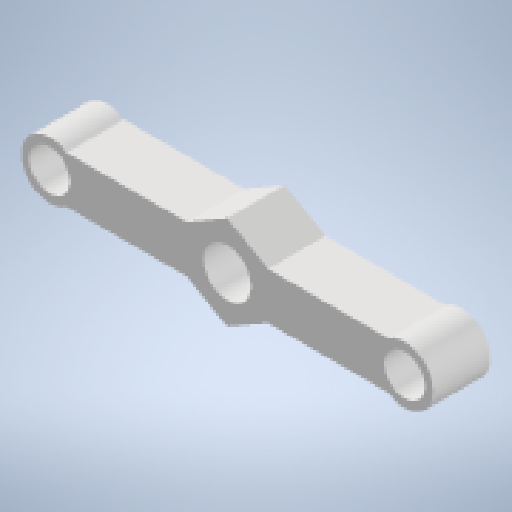
# Autodesk Inventor part: chep_za_os
Saved by Autodesk Inventor 2023 (Build 270158000, 158)
## iProperties
Created: 2022-09-29
Part Number: chep_za_os
Material: Generic
Document SubType Name: Modeling
Designer: simon
Density: 1 g/cm^3
Appearance: Default
Author: simon
Autodesk Inventor part; units mm, degrees
ref_plane "YZ Plane" through (0, 0, 0) normal (1, 0, 0) x (0, 1, 0)
ref_plane "XZ Plane" through (0, 0, 0) normal (0, 1, 0) x (-1, 0, 0)
ref_plane "XY Plane" through (0, 0, 0) normal (0, 0, 1) x (1, 0, 0)
sketch "Sketch1" plane through (0, 0, 0) normal (0, 0, 1) x (1, 0, 0)
  line L0 (0, -7.5) -> (-6.4952, -3.75) projected
  line L1 (-6.4952, -3.75) -> (-6.4952, 3.75) projected
  line L2 (-6.4952, 3.75) -> (0, 7.5) projected
  line L3 (0, 7.5) -> (6.4952, 3.75) projected
  line L4 (6.4952, 3.75) -> (6.4952, -3.75) projected
  line L5 (6.4952, -3.75) -> (0, -7.5) projected
  line L6 (-2.5, -8.366) -> (-2.5, -24.8094) projected
  line L7 (-2.5, -24.8094) -> (-10, -24.8094) projected
  line L8 (-10, -24.8094) -> (-10, -27.8094) projected
  line L9 (10, -27.8094) -> (-10, -27.8094) projected
  line L10 (10, -24.8094) -> (10, -27.8094) projected
  line L11 (10, -24.8094) -> (2.5, -24.8094) projected
  line L12 (2.5, -24.8094) -> (2.5, -8.366) projected
  line L13 (2.5, -8.366) -> (8.4952, -4.9047) projected
  line L14 (8.4952, -4.9047) -> (33.544, -4.9047) projected
  arc A0 (33.544, -4.9047) -> (33.544, 4.9047) centre (37, 0) ccw projected
  line L15 (33.544, 4.9047) -> (8.4952, 4.9047) projected
  line L16 (8.4952, 4.9047) -> (0, 9.8094) projected
  line L17 (0, 9.8094) -> (-8.4952, 4.9047) projected
  line L18 (-8.4952, 4.9047) -> (-33.544, 4.9047) projected
  arc A1 (-33.544, 4.9047) -> (-33.544, -4.9047) centre (-37, 0) ccw projected
  line L19 (-33.544, -4.9047) -> (-8.4952, -4.9047) projected
  line L20 (-8.4952, -4.9047) -> (-2.5, -8.366) projected
  circle A2 centre (37, 0) radius 4.25 projected
  circle A3 centre (-19.7476, 0) radius 2.5 projected
  circle A4 centre (19.7476, 0) radius 2.5 projected
  circle A5 centre (-37.0722, -0.0001) radius 4.25 projected
  line L21 (6.4952, 3.75) -> (6.4952, -3.75) projected
  line L22 (0, 7.5) -> (6.4952, 3.75) projected
  line L23 (-6.4952, 3.75) -> (0, 7.5) projected
  line L24 (-6.4952, -3.75) -> (-6.4952, 3.75) projected
  line L25 (0, -7.5) -> (-6.4952, -3.75) projected
  line L26 (6.4952, -3.75) -> (0, -7.5) projected
  circle A6 centre (0, 0) radius 5 projected
  line L27 (0, 9.8094) -> (8.4952, 4.9047)
  line L28 (8.4952, 4.9047) -> (8.4952, -4.9047)
  line L29 (8.4952, -4.9047) -> (0, -9.8094)
  line L30 (0, -9.8094) -> (-8.4952, -4.9047)
  line L31 (-8.4952, -4.9047) -> (-8.4952, 4.9047)
  line L32 (-8.4952, 4.9047) -> (0, 9.8094)
  constraints: 12 end point, 1 coincident, 13 other
extrude "Extrusion1" add sketch "Sketch1" against normal blind 2 contours L0 L1 L2 L3 L4 L5 | L20 L31 L17 L16 L28 L13 L29 L30 | L19 A1 L18 L31 | L28 L15 A0 L14 | A2 | A3 | A4 | A5
extrude "Extrusion2" add sketch "Sketch1" along normal blind 10 contours L0 L1 L2 L3 L4 L5 | L20 L31 L17 L16 L28 L13 L29 L30 | L19 A1 L18 L31 | L28 L15 A0 L14 | A3 | A4
body "Solid1"
